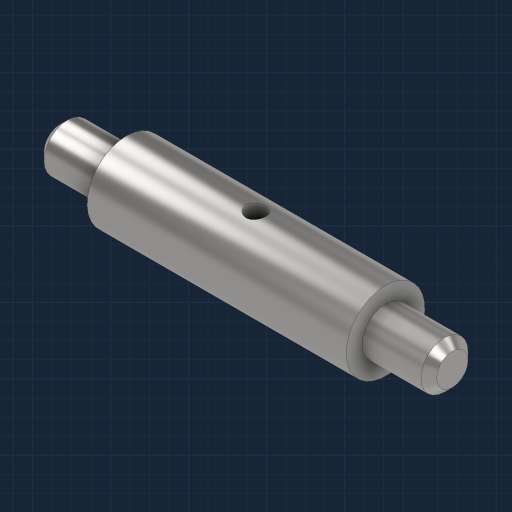
# Autodesk Inventor part: 05-spindel
Saved by Autodesk Inventor 2024 (Build 280153000, 153)
## iProperties
Created: 2025-03-09
Part Number: 05-spindel
Material: Stainless Steel
Document SubType Name: Modeling
Designer: DuctopwH
Density: 8 g/cm^3
Appearance: Semi-Polished
Author: DuctopwH
Autodesk Inventor part; units mm, degrees
ref_plane "YZ Plane" through (0, 0, 0) normal (1, 0, 0) x (0, 1, 0)
ref_plane "XY Plane" through (0, 0, 0) normal (0, 0, 1) x (1, 0, 0)
sketch "Sketch1" plane through (0, 0, 0) normal (0, 0, 1) x (1, 0, 0)
  line L0 (-50, 0) -> (0, 0)
  line L1 (0, 0) -> (50, 0)
  line L2 (-50, 0) -> (-50, 6)
  line L3 (-50, 6) -> (-33, 6)
  line L4 (-33, 6) -> (-33, 10)
  line L5 (-33, 10) -> (33, 10)
  line L6 (33, 10) -> (33, 6)
  line L7 (33, 6) -> (50, 6)
  line L8 (50, 6) -> (50, 0)
  point P0 (-33, 8)
  dimension "d0" = 100
  dimension "d1" = 12
  dimension "d2" = 20
  dimension "d3" = 17
  dimension "d4" = 83
  constraints: 18 end point, 6 perpendicular, 2 collinear, 1 horizontal, 1 midpoint, 1 point on line, 1 vertical
  measures "d0" distance between parallel lines of L2 L8
  measures "d1" diameter of L3 L0
  measures "d2" diameter of L5 L0
  measures "d3" distance from line of point (-33, 8) L2
  measures "d4" distance between parallel lines of L6 L2
revolve "Revolution1" add sketch "Sketch1" angle 360 about axis through (-50, 0, 0) along (1, 0, 0)
sketch "Sketch2" plane through (-50, 0, 0) normal (-1, 0, 0) x (0, 0, 1)
  circle A0 centre (0, 0) radius 6 projected
  constraints: 1 coincident
hole "Hole1" at (-50, 0, 0) direction (1, 0, 0) diameter 5.1 depth 50 tip angle 118
ref_plane "Work Plane1" through (0, 10, 0) normal (0, 1, 0) x (-1, 0, 0)
sketch "Sketch3" plane through (0, 10, 0) normal (0, 1, 0) x (-1, 0, 0)
  line L0 (50, 6) -> (50, -6) projected
  point P0 (0, 0)
  point P1 (0, 0)
  dimension "d13" = 50
  constraints: 1 coincident
  measures "d13" distance from line of L0 point (0, 0)
hole "Hole2" at (0, 10, 0) direction (0, -1, 0) diameter 5.1 depth 14 tip angle 118
chamfer "Chamfer1" distance 2 angle 45 2 edges at (-50, -6, 0) (50, -6, 0)
body "Solid1"
